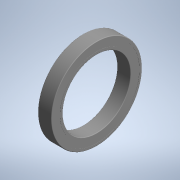
# Autodesk Inventor part: 조인트4베어링
Saved by Autodesk Inventor 2020 (Build 240168000, 168)
## iProperties
Part Number: 조인트4베어링
Material: 일반
Catalog Web Link: www.cadenas.de
Description: B6_ _ _ZZ, SB6_ _ _ZZ-Deep Groove Ball Bearings - Double Shield Type
Vendor: MISUMI
Document SubType Name: Modeling
Designer: partserver
Manufacturer: MISUMI
Mass: 5.3352 g
Surface Area: 33.2418 cm^2
Volume: 5.3352 cm^3
Density: 1 g/cm^3
Appearance: PSOLRGB-175-175-175
Category: PARTsolutions
Company: MISUMI
PSOL_IDENT_0: {$CADENAS_DATA\23d-libs\misumi\metric\12_bearing_holders\sb6010zz.prj},172 {VTYP=3D},{NB=B6807ZZ},{L
PSOL_IDENT_1: INA=B6807ZZ},{NN=B6_ _ _ZZ, SB6_ _ _ZZ},{DATE=30.06.2021 12:59:24},{GEOMDATE=22.10.2019 06:26:04},{V
PSOL_IDENT_2: ERSION=},{LINEID=330},{WBVAR=TS},{WBNUMERIC=}  {NB=B6807ZZ},{LINA=B6807ZZ},{KT=DUMMY},{PN=B6807ZZ},{
PSOL_IDENT_3: TS=},{TS1= '', 'Steel', 'S', 'Stainless Steel'},{MAT=52100 Bearing Steel},{BN=6807ZZ},{DD=35},{D=47}
PSOL_IDENT_4: ,{B=7},{RR=0.3},{CR=4.90},{COR=4.05},{CRS=4.90},{CRSS=4.02},{CORS=4.05},{CORSS=3.06},{DD1=1.00},{R1=
PSOL_IDENT_5: 1.00},{R2=1.0},{DSMIN=37.0},{DSMAX=38.00},{DS1=38.00},{DDHH=45.0},{R=0.3},{MASS=29},{MASS11=29},{AA=
PSOL_IDENT_6: 6.8390},{BB=1.3900},{CC=1.5000},{TYS=w/o Retaining Ring}
NB: B6807ZZ
NN: B6_ _ _ZZ, SB6_ _ _ZZ
NT: Deep Groove Ball Bearings - Double Shield Type
NBSYN: $PN.
LINA: B6807ZZ
CATALOG: Misumi
PN: B6807ZZ
TS: Steel
MAT: 52100 Bearing Steel
BN: 6807ZZ
DD: 35
D: 47
B: 7
RR: 0.3
CR: 4.90
COR: 4.05
DSMIN: 37
DSMAX: 38
DDHH: 45
R: 0.3
MASS: 29
SUPPLIER: MISUMI
ARTICLENO: B6807ZZ
BOMINFO: B6807ZZ
CREATOR: CADENAS GmbH
Title: B6807ZZ
Author: Cadenas PARTsolutions
Comments: Deep Groove Ball Bearings - Double Shield Type
Autodesk Inventor part; units mm, degrees
sketch "Sketch_1" plane through (0, 0, 0) normal (0, 0, 1) x (1, 0, 0)
  line L0 (7, 0) -> (0, 0)
  arc A0 (0, 17.8) -> (0.3, 17.5) centre (0.3, 17.8) ccw
  line L1 (0.3, 17.5) -> (6.7, 17.5)
  arc A1 (6.7, 17.5) -> (7, 17.8) centre (6.7, 17.8) ccw
  line L2 (7, 17.8) -> (7, 19)
  line L3 (7, 19) -> (6.9195, 19)
  line L4 (6.9195, 19) -> (6.9195, 22.11)
  line L5 (6.9195, 22.11) -> (7, 22.11)
  line L6 (7, 22.11) -> (7, 23.2)
  arc A2 (7, 23.2) -> (6.7, 23.5) centre (6.7, 23.2) ccw
  line L7 (6.7, 23.5) -> (0.3, 23.5)
  arc A3 (0.3, 23.5) -> (0, 23.2) centre (0.3, 23.2) ccw
  line L8 (0, 23.2) -> (0, 22.11)
  line L9 (0, 22.11) -> (0.0805, 22.11)
  line L10 (0.0805, 22.11) -> (0.0805, 19)
  line L11 (0.0805, 19) -> (0, 19)
  line L12 (0, 19) -> (0, 17.8)
  constraints: 26 end point, 8 point on circle, 4 centre point
revolve "Revolution1" add sketch "Sketch_1" angle 360 about axis through (7, 0, 0) along (1, 0, 0)
ref_plane "center_point_XY" through (3.5, 0, 0) normal (1, 0, 0) x (0, 0, -1)
ref_plane "center_point_YZ" through (3.5, 0, 0) normal (0, 0, -1) x (0, 1, 0)
ref_plane "center_point_ZX" through (3.5, 0, 0) normal (0, 1, 0) x (1, 0, 0)
ref_plane "to_housing_XY" through (0, 0, 0) normal (1, 0, 0) x (0, 0, -1)
ref_plane "to_housing_YZ" through (0, 0, 0) normal (0, 0, -1) x (0, 1, 0)
ref_plane "to_housing_ZX" through (0, 0, 0) normal (0, 1, 0) x (1, 0, 0)
ref_plane "to_ring_XY" through (6.839, 0, 0) normal (1, 0, 0) x (0, 0, -1)
ref_plane "to_ring_YZ" through (6.839, 0, 0) normal (0, 0, -1) x (0, 1, 0)
ref_plane "to_ring_ZX" through (6.839, 0, 0) normal (0, 1, 0) x (1, 0, 0)
body "Solid1"
